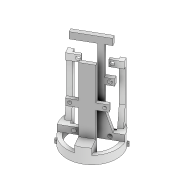
# Autodesk Inventor part: Sujeccion_PCBs
Saved by Autodesk Inventor 2022.3 (Build 263350000, 350)
## iProperties
Created: 2023-07-18
Part Number: Sujeccion_PCBs
Material: Genérico
Document SubType Name: Modeling
Designer: Usuario
Density: 1 g/cm^3
Appearance: Valor por defecto
Author: Usuario
Autodesk Inventor part; units mm, degrees
ref_plane "YZ Plane" through (0, 0, 0) normal (1, 0, 0) x (0, 1, 0)
ref_plane "XZ Plane" through (0, 0, 0) normal (0, 1, 0) x (-1, 0, 0)
ref_plane "XY Plane" through (0, 0, 0) normal (0, 0, 1) x (1, 0, 0)
sketch "Boceto1" plane through (0, 0, 0) normal (0, 1, 0) x (-1, 0, 0)
  arc A0 (-14.0673, -14.2166) -> (-10.4918, -17.0271) centre (0, 0) ccw
  line L0 (1.1244, -10.3205) -> (-10.4918, -17.0271)
  line L1 (1.6244, -11.1865) -> (1.1244, -10.3205)
  line L2 (19.9915, -0.5822) -> (1.6244, -11.1865)
  arc A1 (19.9915, -0.5822) -> (19.8537, 2.4146) centre (0, 0) ccw
  line L3 (20.8464, 2.5353) -> (19.8537, 2.4146)
  arc A2 (20.8464, 2.5353) -> (15.7326, 13.9099) centre (0, 0) ccw
  line L4 (15.7326, 13.9099) -> (14.6319, 13.6347)
  arc A3 (14.6319, 13.6347) -> (-19.8205, -2.6736) centre (0, 0) ccw
  line L5 (-20.7178, -3.431) -> (-19.8205, -2.6736)
  arc A4 (-20.7178, -3.431) -> (-14.9337, -14.7643) centre (0, 0) ccw
  line L6 (-14.9337, -14.7643) -> (-14.0673, -14.2166)
  line L7 (19.1288, 5.8387) -> (20.1107, 6.0466)
  arc A5 (20.1107, 6.0466) -> (-20.7178, -3.431) centre (0, 0) ccw
  line L8 (-20.7178, -3.431) -> (-19.8205, -2.6736)
  arc A6 (19.1288, 5.8387) -> (-19.8205, -2.6736) centre (0, 0) ccw
  line L9 (20.8464, 2.5353) -> (19.8537, 2.4146)
  arc A7 (19.9915, -0.5822) -> (19.8537, 2.4146) centre (0, 0) ccw
  line L10 (19.9915, -0.5822) -> (21, 0)
  arc A8 (21, 0) -> (20.8464, 2.5353) centre (0, 0) ccw
  line L11 (-18.8764, -6.6092) -> (-19.6914, -7.2971)
  arc A9 (-19.6914, -7.2971) -> (-10.5, -18.1865) centre (0, 0) ccw
  line L12 (-10.5, -18.1865) -> (1.6244, -11.1865)
  line L13 (1.6244, -11.1865) -> (1.1244, -10.3205)
  line L14 (1.1244, -10.3205) -> (-10.4918, -17.0271)
  arc A10 (-18.8764, -6.6092) -> (-10.4918, -17.0271) centre (0, 0) ccw
  circle A11 centre (0, 0) radius 19.75
  line L15 (1.1244, -10.3205) -> (0.9994, -10.104)
  line L16 (0.9994, -10.104) -> (-10.4871, -16.7357)
  line L17 (0.9994, -10.104) -> (19.7371, 0.7142)
  circle A12 centre (0, 0) radius 16.75
  line L18 (0.9994, -10.104) -> (0.4994, -9.238)
  line L19 (0.4994, -9.238) -> (-8.4018, -14.4904)
  point P0 (16.552, -2.5681)
  point P1 (19.7365, -0.7295)
  dimension "d2" = 33.5
  dimension "d0" = 39.5
  dimension "d1" = 0.25
  dimension "d3" = 1
  constraints: 40 end point, 24 point on circle, 12 centre point, 2 coincident, 2 perpendicular, 1 point on line, 3 other
  measures "d0" diameter of A11
  measures "d1" distance of L13.end L15.end
  measures "d3" distance of L15.end L18.end
extrude "Extrusión1" add sketch "Boceto1" along normal blind 6.5 contours A11 L17 A12 L16 | A12 L19 L18 L16 | A11 L2 A12 L17
sketch "Boceto2" plane through (0, 0, 0) normal (0, 1, 0) x (-1, 0, 0)
  arc A0 (14.6319, 13.6347) -> (-19.8205, -2.6736) centre (0, 0) ccw
  arc A1 (19.1288, 5.8387) -> (-19.8205, -2.6736) centre (0, 0) ccw
  arc A2 (20.1107, 6.0466) -> (-20.7178, -3.431) centre (0, 0) ccw
  line L0 (19.9915, -0.5822) -> (1.6244, -11.1865)
  line L1 (15.7326, 13.9099) -> (14.6319, 13.6347)
  arc A3 (19.9915, -0.5822) -> (19.8537, 2.4146) centre (0, 0) ccw
  arc A4 (19.9915, -0.5822) -> (19.8537, 2.4146) centre (0, 0) ccw
  line L2 (19.9915, -0.5822) -> (21, 0)
  arc A5 (21, 0) -> (20.8464, 2.5353) centre (0, 0) ccw
  line L3 (19.1288, 5.8387) -> (20.1107, 6.0466)
  line L4 (20.8464, 2.5353) -> (19.8537, 2.4146)
  line L5 (20.8464, 2.5353) -> (19.8537, 2.4146)
  arc A6 (20.8464, 2.5353) -> (15.7326, 13.9099) centre (0, 0) ccw
  line L6 (1.6244, -11.1865) -> (1.1244, -10.3205)
  arc A7 (-14.0673, -14.2166) -> (-10.4918, -17.0271) centre (0, 0) ccw
  line L7 (1.1244, -10.3205) -> (-10.4918, -17.0271)
  arc A8 (-20.7178, -3.431) -> (-14.9337, -14.7643) centre (0, 0) ccw
  line L8 (-14.9337, -14.7643) -> (-14.0673, -14.2166)
  line L9 (-18.8764, -6.6092) -> (-19.6914, -7.2971)
  line L10 (1.6244, -11.1865) -> (1.1244, -10.3205)
  arc A9 (-18.8764, -6.6092) -> (-10.4918, -17.0271) centre (0, 0) ccw
  arc A10 (-19.6914, -7.2971) -> (-10.5, -18.1865) centre (0, 0) ccw
  line L11 (1.1244, -10.3205) -> (-10.4918, -17.0271)
  line L12 (-10.5, -18.1865) -> (1.6244, -11.1865)
  line L13 (-20.7178, -3.431) -> (-19.8205, -2.6736)
  line L14 (-20.7178, -3.431) -> (-19.8205, -2.6736)
  circle A11 centre (0, 0) radius 19.75
  line L15 (1.1244, -10.3205) -> (0.9994, -10.104)
  line L16 (0.9994, -10.104) -> (-10.4871, -16.7357)
  line L17 (0.9994, -10.104) -> (19.7371, 0.7142)
  circle A12 centre (0, 0) radius 16.75
  line L18 (0.9994, -10.104) -> (0.4994, -9.238)
  line L19 (0.4994, -9.238) -> (-8.4018, -14.4904)
  line L20 (-14.9337, -14.7643) -> (-13.8504, -14.0794)
  arc A13 (19.7365, -0.7295) -> (-10.4871, -16.7357) centre (0, 0) ccw projected
  line L21 (-16.2705, -13.2767) -> (-15.2057, -12.6035)
  line L22 (14.6319, 13.6347) -> (14.3543, 13.5653)
  line L23 (16.9845, 12.3502) -> (15.8956, 11.7215)
  point P0 (16.552, -2.5681)
  dimension "d8" = 33.5
  dimension "d6" = 39.5
  dimension "d7" = 0.25
  dimension "d9" = 1
  dimension "d10" = 2
  dimension "d11" = 2
  constraints: 48 end point, 30 point on circle, 12 centre point, 2 coincident, 2 perpendicular, 2 point on line, 1 parallel, 3 other
  measures "d6" diameter of A11
  measures "d7" distance of L10.end L15.end
  measures "d9" distance of L15.end L18.end
  measures "d10" distance of L8.start L21.start
  measures "d11" distance of L1.start L23.start
extrude "Extrusión2" add sketch "Boceto2" along normal blind 2.4 contours L1 A2 L23 A1 | A1 L23 A11 L22 | A11 L20 A9 L21 | A9 L8 A8 L21
sketch "Boceto3" plane through (-0.9994, 0, -10.104) normal (-0.5, 0, -0.8660254) x (-0.8660254, 0, 0.5)
  line L0 (0, 0) -> (0, 6.5) projected
  line L1 (0, 3.25) -> (-7, 3.25)
  circle A0 centre (-7, 3.25) radius 1.5
  point P0 (4.1865, 0)
  dimension "d14" = 7
  dimension "d15" = 3
  constraints: 2 end point, 1 centre point, 1 coincident, 1 horizontal, 1 midpoint
  measures "d14" distance of L1.start L1.end
  measures "d15" diameter of A0
extrude "Extrusión3" cut sketch "Boceto3" against normal blind 1
sketch "Boceto5" plane through (0, 6.5, 0) normal (0, 1, 0) x (1, 0, 0)
  arc A0 (-19.7365, 0.7295) -> (10.4871, 16.7357) centre (0, 0) ccw projected
  circle A1 centre (0, 0) radius 19.75
  arc A2 (-16.552, 2.5681) -> (8.4018, 14.4904) centre (0, 0) ccw projected
  circle A3 centre (0, 0) radius 16.75
  line L0 (-16.552, 2.5681) -> (-19.7365, 0.7295) projected
  line L1 (-16.552, 2.5681) -> (-19.7365, 0.7295)
  line L2 (10.4871, 16.7357) -> (7.4684, 14.9929)
  line L3 (10.4871, 16.7357) -> (-0.9994, 10.104) projected
  line L4 (-0.9994, 10.104) -> (8.0006, -5.4845)
  line L5 (8.0006, -5.4845) -> (6.5006, -2.8864)
  line L6 (6.5006, -2.8864) -> (16.4994, 2.8864)
  line L7 (6.5006, -2.8864) -> (-10.7494, -12.8457)
  line L8 (7.4684, 14.9929) -> (14.9684, 2.0025)
  line L9 (-16.552, 2.5681) -> (-8.427, -11.5048)
  line L10 (8.0006, -5.4845) -> (19.7088, 1.2752)
  line L11 (8.0006, -5.4845) -> (-10.9588, -16.4307)
  point P0 (19.7088, 1.2752)
  point P1 (-10.9588, -16.4307)
  dimension "d18" = 18
  dimension "d22" = 3
  constraints: 20 end point, 7 point on circle, 6 point on line, 2 centre point, 2 coincident, 2 perpendicular, 1 collinear
  measures "d18" distance of L3.end L4.end
  measures "d22" distance of L4.end L5.end
extrude "Extrusión4" add sketch "Boceto5" along normal blind 5 contours L0 A2 L11 A0 | A0 L10 A2 A3 L2 | L9 L7 A2 | A2 L7 L4 L11 | A3 A2 L6 L8 | L10 L4 L6 A2
sketch "Boceto7" plane through (0, 11.5, 0) normal (0, 1, 0) x (1, 0, 0)
  line L0 (7.4684, 14.9929) -> (14.9684, 2.0025) projected
  line L1 (7.4684, 14.9929) -> (8.4684, 13.2608)
  arc A0 (19.7088, 1.2752) -> (10.4871, 16.7357) centre (0, 0) ccw projected
  line L2 (10.4871, 16.7357) -> (11.4871, 15.0036)
  line L3 (8.4684, 13.2608) -> (11.4871, 15.0036)
  line L4 (7.922, 14.2073) -> (14.9684, 2.0025) projected
  line L5 (-16.552, 2.5681) -> (-19.7365, 0.7295) projected
  line L6 (-16.552, 2.5681) -> (-14.927, -0.2465)
  line L7 (-8.427, -11.5048) -> (-16.552, 2.5681) projected
  line L8 (-19.7365, 0.7295) -> (-18.1115, -2.0851)
  line L9 (-18.1115, -2.0851) -> (-14.927, -0.2465)
  line L10 (10.4871, 16.7357) -> (7.4684, 14.9929)
  line L11 (10.4871, 16.7357) -> (-0.9994, 10.104) projected
  dimension "d23" = 2
  constraints: 14 end point, 3 point on line, 2 perpendicular, 1 collinear, 1 parallel
  measures "d23" distance of L0.start L1.end
extrude "Extrusión5" add sketch "Boceto7" along normal blind 45
chamfer "Chaflán1" distance 14 angle 15 1 edges at (9.9777, 11.5, -14.1322) measured on face at (9.9777, 12, -14.1322)
chamfer "Chaflán2" distance 14 angle 15 1 edges at (-16.5192, 11.5, 1.1658) measured on face at (-16.5192, 12, 1.1658)
sketch "Boceto8" plane through (0, 56.5, 0) normal (0, 1, 0) x (1, 0, 0)
  line L0 (11.4871, 15.0036) -> (8.4684, 13.2608) projected
  line L1 (11.4871, 15.0036) -> (12.4871, 13.2716)
  line L2 (12.4871, 13.2716) -> (9.4684, 11.5288)
  line L3 (7.922, 14.2073) -> (14.9684, 2.0025) projected
  line L4 (9.4684, 11.5288) -> (8.4684, 13.2608)
  line L5 (8.4684, 13.2608) -> (11.4871, 15.0036)
  line L6 (12.4871, 13.2716) -> (4.6929, 8.7716)
  line L7 (4.6929, 8.7716) -> (3.6929, 10.5036)
  line L8 (3.6929, 10.5036) -> (8.4684, 13.2608)
  line L9 (-16.2359, -5.3338) -> (-19.7365, 0.7295) projected
  line L10 (-18.1115, -2.0851) -> (-17.1115, -3.8172)
  line L11 (-17.1115, -3.8172) -> (-9.3173, 0.6828)
  line L12 (-9.3173, 0.6828) -> (-10.3173, 2.4149)
  line L13 (-14.927, -0.2465) -> (-18.1115, -2.0851) projected
  line L14 (-10.3173, 2.4149) -> (-18.1115, -2.0851)
  point P0 (0, 0)
  dimension "d32" = 2
  dimension "d33" = 9
  dimension "d34" = 9
  constraints: 22 end point, 7 point on line, 6 perpendicular, 1 collinear, 1 parallel
  measures "d32" distance of L0.start L1.end
  measures "d33" distance of L1.end L6.end
  measures "d34" distance of L10.end L11.end
extrude "Extrusión6" add sketch "Boceto8" against normal blind 5
sketch "Boceto9" plane through (8.4684, 51.5, -13.2608) normal (-0.5, 0, -0.8660254) x (-0.8660254, 0, 0.5)
  line L0 (0, -45) -> (0, 5) projected
  line L1 (0, 5) -> (0, 0)
  line L2 (-3.4857, 0) -> (5.5143, 0) projected
  line L3 (0, 2.5) -> (27.0146, 2.5)
  line L4 (27.0146, -45) -> (27.0146, 5) projected
  line L5 (13.5073, 2.5) -> (3.5073, 2.5)
  line L6 (13.5073, 2.5) -> (23.5073, 2.5)
  circle A0 centre (3.5073, 2.5) radius 1.5
  circle A1 centre (23.5073, 2.5) radius 1.5
  point P0 (13.9642, -51.5)
  dimension "d37" = 10
  dimension "d38" = 10
  dimension "d39" = 3
  dimension "d40" = 3
  constraints: 8 end point, 4 point on line, 2 centre point, 2 coincident, 2 midpoint, 1 perpendicular, 1 vertical
  measures "d37" distance of L5.start L5.end
  measures "d38" distance of L5.start L6.end
  measures "d39" diameter of A0
  measures "d40" diameter of A1
extrude "Extrusión7" cut sketch "Boceto9" against normal through all
sketch "Boceto10" plane through (0, 11.5, 0) normal (0, 1, 0) x (1, 0, 0)
  line L0 (19.7088, 1.2752) -> (11.0485, -3.7248)
  line L1 (-7.9943, -14.7192) -> (16.7443, -0.4363) projected
  line L2 (11.0485, -3.7248) -> (9.5485, -1.1267)
  line L3 (9.5485, -1.1267) -> (6.0844, -3.1267)
  line L4 (14.9684, 2.0025) -> (-8.427, -11.5048) projected
  line L5 (6.0844, -3.1267) -> (7.5844, -5.7248)
  line L6 (7.5844, -5.7248) -> (11.0485, -3.7248)
  point P0 (0, 0)
  dimension "d43" = 10
  dimension "d44" = 4
  constraints: 10 end point, 3 perpendicular, 3 point on line
  measures "d43" distance of L0.start L0.end
  measures "d44" distance of L2.end L3.end
extrude "Extrusión8" add sketch "Boceto10" along normal blind 75
sketch "Boceto11" plane through (9.5485, 11.5, 1.1267) normal (0.8660254, 0, -0.5) x (-0.5, 0, -0.8660254)
  line L0 (-3, 75) -> (0, 75) projected
  line L1 (-3, 0) -> (-3, 75) projected
  line L2 (0, 75) -> (-3, 75)
  line L3 (-3, 75) -> (-3, 70)
  line L4 (-3, 70) -> (0, 70)
  line L5 (0, 70) -> (0, 75)
  point P0 (5.75, -11.5)
  dimension "d47" = 5
  constraints: 8 end point, 2 parallel, 1 horizontal, 1 perpendicular, 1 point on line
  measures "d47" distance of L3.end L2.end
extrude "Extrusión9" add sketch "Boceto11" along normal blind 6
sketch "Boceto12" plane through (7.5844, 11.5, 5.7248) normal (-0.8660254, 0, 0.5) x (0.5, 0, 0.8660254)
  line L0 (-3, 75) -> (0, 75) projected
  line L1 (0, 75) -> (0, 70) projected
  line L2 (0, 70) -> (-3, 70) projected
  line L3 (-3, 70) -> (-3, 75) projected
  point P0 (-8.75, -11.5)
extrude "Extrusión10" add sketch "Boceto12" along normal blind 16.5
sketch "Boceto13" plane through (19.7088, 6.5, -1.2752) normal (0.5, 0, 0.8660254) x (0.8660254, 0, -0.5)
  line L0 (-30.5, 80) -> (-30.5, 75) projected
  line L1 (-30.5, 77.5) -> (-4, 77.5)
  line L2 (-4, 80) -> (-4, 75) projected
  line L3 (-17.25, 77.5) -> (-27.75, 77.5)
  line L4 (-17.25, 77.5) -> (-6.75, 77.5)
  circle A0 centre (-27.75, 77.5) radius 1.5
  circle A1 centre (-6.75, 77.5) radius 1.5
  point P0 (-17.7059, -6.5)
  dimension "d52" = 10.5
  dimension "d53" = 10.5
  dimension "d54" = 3
  dimension "d55" = 3
  constraints: 6 end point, 3 midpoint, 2 centre point, 2 coincident, 2 point on line
  measures "d52" distance of L3.start L3.end
  measures "d53" distance of L3.start L4.end
  measures "d54" diameter of A0
  measures "d55" diameter of A1
extrude "Extrusión11" cut sketch "Boceto13" against normal through all
sketch "Boceto14" plane through (19.7088, 6.5, -1.2752) normal (0.5, 0, 0.8660254) x (0.8660254, 0, -0.5)
  line L0 (-10, 5) -> (-10, 75) projected
  line L1 (-10, 75) -> (-10, 42.7)
  line L2 (-10, 42.7) -> (-4, 42.7)
  line L3 (-3.7417, 0) -> (-3.7417, 50) projected
  line L4 (-4, 42.7) -> (-4, 37.7)
  line L5 (-4, 42.7) -> (1, 42.7) construction
  line L6 (-4, 37.7) -> (-10, 37.7)
  line L7 (-10, 37.7) -> (-10, 42.7)
  circle A0 centre (-6.75, 77.5) radius 1.5 projected
  line L8 (-6.75, 77.5) -> (-6.75, 40.2)
  circle A1 centre (-6.75, 40.2) radius 1.5
  point P0 (-17.7059, -6.5)
  dimension "d58" = 32.3
  dimension "d59" = 6
  dimension "d60" = 5
  dimension "d61" = 90
  dimension "d65" = 37.3
  dimension "d66" = 3
  constraints: 14 end point, 3 perpendicular, 2 point on line, 1 centre point, 1 coincident, 1 collinear, 1 horizontal, 1 vertical
  measures "d58" distance of L0.end L1.end
  measures "d59" distance of L1.end L2.end
  measures "d60" distance of L2.end L4.end
  measures "d61" angle of L4 L5
  measures "d65" distance of L8.start L8.end
  measures "d66" diameter of A1
extrude "Extrusión12" add sketch "Boceto14" against normal blind 3 contours L0 L2 L4 L6
sketch "Boceto17" plane through (19.7088, 6.5, -1.2752) normal (0.5, 0, 0.8660254) x (0.8660254, 0, -0.5)
  line L0 (0, 0) -> (-35.4119, 0) projected
  line L1 (0, 0) -> (12.1594, 0)
  line L2 (12.1594, 0) -> (-50.5661, 0)
  line L3 (-50.5661, 0) -> (-50.5661, 87.0058)
  line L4 (-50.5661, 87.0058) -> (12.1594, 87.0058)
  line L5 (12.1594, 87.0058) -> (12.1594, 0)
  point P0 (-17.7059, -6.5)
  constraints: 10 end point, 2 horizontal, 2 parallel, 1 perpendicular
extrude "Extrusión13" cut sketch "Boceto17" against normal blind 7
sketch "Boceto18" plane through (16.2088, 6.5, -7.3374) normal (0.5, 0, 0.8660254) x (0.8660254, 0, -0.5)
  line L0 (-37.3782, 5) -> (1.9664, 5) projected
  line L1 (1.9664, 0) -> (-1.0476, 0) projected
  line L2 (-37.3782, 5) -> (1.9664, 5)
  line L3 (1.9664, 5) -> (1.9664, 0)
  line L4 (1.9664, 0) -> (-37.3782, 0)
  line L5 (-37.3782, 0) -> (-37.3782, 5)
  point P0 (-17.7059, -6.5)
  point P1 (-30.7563, 5)
  point P2 (-30.7563, 5)
  constraints: 8 end point, 2 parallel, 1 horizontal, 1 perpendicular
extrude "Extrusión14" add sketch "Boceto18" against normal blind 3
sketch "Boceto20" plane through (14.7088, 6.5, -9.9355) normal (-0.5, 0, -0.8660254) x (-0.8660254, 0, 0.5)
  line L0 (-1.6454, 0) -> (-1.6454, 5)
  line L1 (-1.6454, 2.5) -> (1.1885, 2.5)
  line L2 (1.1885, 5) -> (1.1885, 0)
  line L3 (17.249, 2.5) -> (17.249, 5)
  line L4 (4.1986, 5) -> (-3.7417, 5)
  line L5 (30.499, 5) -> (30.499, 0)
  line L6 (17.249, 2.5) -> (17.249, 0)
  circle A0 centre (27.749, 2.5) radius 1.5
  line L7 (3.999, 0) -> (3.999, 5)
  circle A1 centre (6.749, 2.5) radius 1.5
  line L8 (9.999, 5) -> (3.999, 5)
  line L9 (3.999, 2.5) -> (-4.4559, 2.5)
  line L10 (3.999, 0) -> (30.499, 0)
  line L11 (13.999, 5) -> (30.499, 5)
  line L12 (9.999, 37.3) -> (9.999, 5)
  line L13 (3.999, 37.3) -> (9.999, 37.3)
  circle A2 centre (6.749, 39.8) radius 1.5
  line L14 (3.999, 42.3) -> (3.999, 37.3)
  line L15 (9.999, 42.3) -> (3.999, 42.3)
  line L16 (9.999, 65) -> (4.999, 65)
  line L17 (37.3782, 5) -> (-1.9664, 5) projected
  line L18 (1.0476, 0) -> (34.3643, 0) projected
  line L19 (0.256, -6.5) -> (0.256, 5) projected
  line L20 (3.7417, 0) -> (3.7417, 5) projected
  line L21 (3.7417, 2.5) -> (30.7563, 2.5)
  line L22 (30.7563, 5) -> (30.7563, 0) projected
  line L23 (17.249, 2.5) -> (17.249, 5)
  line L24 (30.4109, 65) -> (30.4109, 70)
  line L25 (4.999, 65) -> (4.999, 70)
  line L26 (30.4109, 65) -> (13.999, 65)
  line L27 (30.4109, 70) -> (4.999, 70)
  line L28 (13.999, 65) -> (13.999, 5)
  line L29 (9.999, 65) -> (9.999, 42.3)
  point P0 (17.7059, -6.5)
  point P1 (17.249, -6.5)
  point P2 (14.6875, 2.1)
  point P3 (9.999, 5)
  point P4 (13.999, 5)
  point P5 (9.999, 5)
  point P6 (30.499, 5)
  point P7 (3.999, 5)
  point P8 (9.999, 65)
  point P9 (13.999, 5)
  dimension "d83" = 0
  constraints: 50 end point, 5 midpoint, 3 centre point, 3 perpendicular, 1 parallel, 1 point on line, 1 vertical
  measures "d83" distance of L16.start L29.start
extrude "Extrusión15" add sketch "Boceto20" against normal blind 3 contours L12 L13 L14 L15 L29 L16 L25 L27 L24 L26 L28 L17
sketch "Boceto21" plane through (14.7088, 6.5, -9.9355) normal (-0.5, 0, -0.8660254) x (-0.8660254, 0, 0.5)
  line L0 (-1.6454, 0) -> (-1.6454, 5)
  line L1 (-1.6454, 2.5) -> (1.1885, 2.5)
  line L2 (1.1885, 5) -> (1.1885, 0)
  line L3 (17.249, 2.5) -> (17.249, 5)
  line L4 (4.1986, 5) -> (-3.7417, 5)
  line L5 (30.499, 5) -> (30.499, 0)
  line L6 (17.249, 2.5) -> (17.249, 0)
  circle A0 centre (27.749, 2.5) radius 1.5
  line L7 (3.999, 0) -> (3.999, 5)
  circle A1 centre (6.749, 2.5) radius 1.5
  line L8 (9.999, 5) -> (3.999, 5)
  line L9 (3.999, 2.5) -> (-4.4559, 2.5)
  line L10 (3.999, 0) -> (30.499, 0)
  line L11 (13.999, 5) -> (30.499, 5)
  line L12 (9.999, 37.3) -> (9.999, 5)
  line L13 (3.999, 37.3) -> (9.999, 37.3)
  circle A2 centre (6.749, 39.8) radius 1.5
  line L14 (3.999, 42.3) -> (3.999, 37.3)
  line L15 (9.999, 42.3) -> (3.999, 42.3)
  line L16 (13.999, 75) -> (13.999, 5)
  line L17 (9.999, 75) -> (9.999, 42.3)
  line L18 (35.4109, 80) -> (35.4109, 75)
  line L19 (31.9878, 80) -> (35.4109, 80)
  line L20 (-0.001, 80) -> (-0.001, 75)
  line L21 (-0.001, 80) -> (3.4221, 80)
  line L22 (9.999, 75) -> (-0.001, 75)
  line L23 (31.9878, 80) -> (3.4221, 80)
  line L24 (35.4109, 75) -> (13.999, 75)
  line L25 (36.6004, 5) -> (-1.1885, 5)
  line L26 (1.9738, 0) -> (33.4381, 0)
  line L27 (0.256, -6.5) -> (0.256, 5)
  line L28 (3.7417, 0) -> (3.7417, 5)
  line L29 (3.7417, 2.5) -> (30.7563, 2.5)
  line L30 (30.7563, 5) -> (30.7563, 0)
  line L31 (17.249, 2.5) -> (17.249, 5)
  point P0 (17.7059, -6.5)
  point P1 (17.7059, -6.5)
  point P2 (17.249, -6.5)
  point P3 (14.6875, 2.1)
  point P4 (9.999, 5)
  point P5 (13.999, 5)
  constraints: 64 end point, 5 midpoint, 3 centre point, 1 perpendicular, 1 point on line, 1 vertical
extrude "Extrusión16" cut sketch "Boceto21" against normal blind 3 contours L29 A1 | A1 L29 | L29 A0 | A0 L29
chamfer "Chaflán3" distance 5 distance2 15 1 edges at (3.3353, 11.5, -1.637) measured on face at (2.9023, 11.5, -1.387)
chamfer "Chaflán4" distance 5 distance2 15 1 edges at (6.7994, 11.5, -3.637) measured on face at (7.2324, 11.5, -3.887)
sketch "Boceto22" plane through (0, 6.5, 0) normal (0, 1, 0) x (1, 0, 0)
  line L0 (-11.6278, -5.2699) -> (-10.1278, -7.868) projected
  line L1 (-10.1278, -7.868) -> (12.9684, 5.4666)
  line L2 (11.4684, 8.0647) -> (-11.927, -5.4427) projected
  line L3 (11.8795, 4.8379) -> (-10.1278, -7.868) projected
  line L4 (0.8759, -1.515) -> (3.8759, -6.7112)
  line L5 (0.8759, -1.515) -> (6.8759, -1.515) construction
  line L6 (3.8759, -6.7112) -> (16.7348, 0.7129)
  arc A0 (-13.5515, -9.8447) -> (15.3015, 6.8136) centre (0, 0) ccw projected
  line L7 (16.7348, 0.7129) -> (-8.9848, -14.1363)
  line L8 (3.8759, -6.7112) -> (5.3759, -9.3093)
  line L9 (5.3759, -9.3093) -> (-5.7493, -15.7324)
  line L10 (5.3759, -9.3093) -> (16.4993, -2.8872)
  line L11 (-8.9848, -14.1363) -> (-10.4871, -16.7357)
  arc A1 (-16.1617, -11.3517) -> (17.9117, 8.3206) centre (0, 0) ccw projected
  line L12 (19.7371, 0.7142) -> (16.7348, 0.7129)
  line L13 (3.8759, -6.7112) -> (-0.4543, -9.2112)
  line L14 (-0.4543, -9.2112) -> (5.2242, -19.0465)
  line L15 (3.8759, -6.7112) -> (8.206, -4.2112)
  line L16 (8.206, -4.2112) -> (13.8842, -14.0461)
  point P0 (8.206, -4.2112)
  dimension "d84" = 6
  dimension "d85" = 60
  dimension "d86" = 90
  dimension "d87" = 3
  dimension "d88" = 5
  dimension "d89" = 5
  constraints: 28 end point, 8 point on circle, 5 perpendicular, 4 point on line, 1 equal length, 1 horizontal, 1 midpoint, 1 parallel
  measures "d84" distance of L4.start L4.end
  measures "d85" angle of L4 L5
  measures "d86" angle of L6 L4
  measures "d87" distance of L4.end L8.end
  measures "d88" distance of L4.end L13.end
  measures "d89" distance of L4.end L15.end
extrude "Extrusión17" add sketch "Boceto22" along normal blind 5 contours L8 L9 L14 L7 | L6 L16 L10 L8 | L10 L16 A0 L14 L9 | L16 A1 L14 A0
sketch "Boceto23" plane through (0, 6.5, 0) normal (0, -1, 0) x (1, 0, 0)
  arc A0 (12.324, 11.3438) -> (3.6641, 16.3443) centre (0, 0) ccw projected
  line L0 (-0.4543, 9.2112) -> (3.6641, 16.3443) projected
  line L1 (8.206, 4.2112) -> (-0.4543, 9.2112) projected
  line L2 (12.324, 11.3438) -> (8.206, 4.2112) projected
extrude "Extrusión18" add sketch "Boceto23" along normal blind 6.5
sketch "Boceto24" plane through (0, 11.5, 0) normal (0, 1, 0) x (1, 0, 0)
  line L0 (8.206, -4.2112) -> (-0.4543, -9.2112) projected
  line L1 (-0.4543, -9.2112) -> (8.206, -4.2112)
  line L2 (8.206, -4.2112) -> (9.456, -6.3763)
  line L3 (8.206, -4.2112) -> (12.324, -11.3438) projected
  line L4 (9.456, -6.3763) -> (0.7957, -11.3763)
  line L5 (-0.4543, -9.2112) -> (5.2242, -19.0465) projected
  line L6 (0.7957, -11.3763) -> (-0.4543, -9.2112)
  point P0 (0, 0)
  dimension "d94" = 2.5
  constraints: 8 end point, 2 collinear, 2 point on line, 1 perpendicular
  measures "d94" distance of L0.start L2.end
extrude "Extrusión19" add sketch "Boceto24" along normal blind 51
sketch "Boceto25" plane through (9.456, 11.5, 6.3763) normal (0.5, 0, 0.8660254) x (0.8660254, 0, -0.5)
  line L0 (0, 0) -> (-10, 0) projected
  line L1 (-5, 0) -> (-5, 20)
  line L2 (-5, 20) -> (-5, 22.54)
  line L3 (-5, 22.54) -> (-15.16, 22.54)
  line L4 (-5, 22.54) -> (5.16, 22.54)
  circle A0 centre (5.16, 22.54) radius 1.25
  circle A1 centre (-15.16, 22.54) radius 1.25
  line L5 (-15.16, 22.54) -> (-17.7, 22.54)
  line L6 (-18.0514, -5) -> (-18.0514, 45) projected
  line L7 (5.16, 22.54) -> (7.7, 22.54)
  line L8 (-5, 22.54) -> (-5, 25.08)
  line L9 (-5, 25.08) -> (-17.7, 25.08)
  line L10 (-17.7, 25.08) -> (-17.7, 20)
  line L11 (-17.7, 20) -> (-5, 20)
  line L12 (-5, 20) -> (7.7, 20)
  line L13 (7.7, 20) -> (7.7, 25.08)
  line L14 (7.7, 25.08) -> (-5, 25.08)
  point P0 (-5.001, -11.5)
  dimension "d97" = 20
  dimension "d98" = 2.54
  dimension "d99" = 10.16
  dimension "d100" = 10.16
  dimension "d101" = 2.5
  dimension "d102" = 2.5
  dimension "d103" = 2.54
  dimension "d104" = 2.54
  dimension "d105" = 2.54
  constraints: 26 end point, 7 perpendicular, 3 point on line, 2 centre point, 2 coincident, 2 horizontal, 2 vertical, 1 midpoint
  measures "d97" distance of L1.start L1.end
  measures "d98" distance of L1.end L2.end
  measures "d99" distance of L2.end L3.end
  measures "d100" distance of L2.end L4.end
  measures "d101" diameter of A0
  measures "d102" diameter of A1
  measures "d103" distance of L5.start L5.end
  measures "d104" distance of L7.start L7.end
  measures "d105" distance of L2.end L8.end
extrude "Extrusión20" add sketch "Boceto25" against normal blind 2.5 contours L11 L10 L5 A1 L3 L2 | L2 L4 A0 L7 L13 L12 | L8 L14 L13 L7 A0 L4 | L3 A1 L5 L10 L9 L8
